Autodesk Fusion 360 part; units mm, degrees
(part 3 of 4)
  arc A61 (-18.7401, 17.7754) -> (-17.3539, 17.7855) centre (-18.0523, 18.5012) ccw
  line L30 (-18.7401, 17.7754) -> (-19.4311, 18.4301)
  spline S30 degree 5 poles (-19.4311, 18.4301) (-19.4412, 18.4397) (-19.4617, 18.4586) (-19.4931, 18.486) (-19.5364, 18.521) (-19.5924, 18.5625) (-19.6498, 18.6024) (-19.708, 18.6413) (-19.7667, 18.6797) (-19.8257, 18.7177) (-19.885, 18.7553) (-19.9448, 18.7924) (-20.0051, 18.8288) (-20.0661, 18.8644) (-20.1276, 18.8992) (-20.1898, 18.9332) (-20.2525, 18.9666) (-20.3156, 18.9995) (-20.379, 19.0319) (-20.4428, 19.0638) (-20.5069, 19.0953) (-20.5714, 19.1263) (-20.6362, 19.1568) (-20.7014, 19.1867) (-20.767, 19.2162) (-20.8329, 19.2451) (-20.8992, 19.2736) (-20.9657, 19.3016) (-21.0326, 19.3292) (-21.0998, 19.3564) (-21.1672, 19.3831) (-21.235, 19.4094) (-21.303, 19.4353) (-21.3713, 19.4607) (-21.4399, 19.4857) (-21.5088, 19.5103) (-21.5779, 19.5345) (-21.6473, 19.5583) (-21.7169, 19.5816) (-21.7868, 19.6046) (-21.8569, 19.6271) (-21.9273, 19.6493) (-21.9979, 19.6711) (-22.0687, 19.6925) (-22.1398, 19.7135) (-22.2111, 19.7341) (-22.2826, 19.7543) (-22.3543, 19.7742) (-22.4263, 19.7936) (-22.4985, 19.8127) (-22.5708, 19.8315) (-22.6434, 19.8498) (-22.7162, 19.8678) (-22.7892, 19.8854) (-22.8623, 19.9027) (-22.9357, 19.9195) (-23.0093, 19.9361) (-23.083, 19.9522) (-23.157, 19.968) (-23.2311, 19.9835) (-23.3054, 19.9986) (-23.3799, 20.0133) (-23.4545, 20.0277) (-23.5293, 20.0417) (-23.6043, 20.0554) (-23.6795, 20.0687) (-23.7548, 20.0817) (-23.8303, 20.0943) (-23.906, 20.1066) (-23.9818, 20.1185) (-24.0578, 20.1301) (-24.1187, 20.1391) (-24.1645, 20.1457) (-24.195, 20.1501) (-24.2103, 20.1522) knots 0 0 0 0 0 0 0.01428571 0.02857143 0.04285714 0.05714286 0.07142857 0.08571429 0.1 0.11428571 0.12857143 0.14285714 0.15714286 0.17142857 0.18571429 0.2 0.21428571 0.22857143 0.24285714 0.25714286 0.27142857 0.28571429 0.3 0.31428571 0.32857143 0.34285714 0.35714286 0.37142857 0.38571429 0.4 0.41428571 0.42857143 0.44285714 0.45714286 0.47142857 0.48571429 0.5 0.51428571 0.52857143 0.54285714 0.55714286 0.57142857 0.58571429 0.6 0.61428571 0.62857143 0.64285714 0.65714286 0.67142857 0.68571429 0.7 0.71428571 0.72857143 0.74285714 0.75714286 0.77142857 0.78571429 0.8 0.81428571 0.82857143 0.84285714 0.85714286 0.87142857 0.88571429 0.9 0.91428571 0.92857143 0.94285714 0.95714286 0.97142857 0.98571429 1 1 1 1 1 1
  arc A62 (-24.2103, 20.1522) -> (-25.4788, 18.5224) centre (0, 0) ccw
  spline S31 degree 5 poles (-22.6362, 14.3122) (-22.648, 14.3196) (-22.6713, 14.3348) (-22.7056, 14.3586) (-22.7502, 14.392) (-22.8041, 14.4361) (-22.8569, 14.4819) (-22.9089, 14.5288) (-22.9605, 14.5763) (-23.0118, 14.6241) (-23.0628, 14.6724) (-23.1135, 14.7212) (-23.1636, 14.7708) (-23.213, 14.8211) (-23.2619, 14.8723) (-23.3102, 14.9242) (-23.3579, 14.9767) (-23.4053, 15.0298) (-23.4522, 15.0834) (-23.4989, 15.1374) (-23.5451, 15.1918) (-23.591, 15.2467) (-23.6365, 15.302) (-23.6815, 15.3579) (-23.7262, 15.4142) (-23.7704, 15.471) (-23.8143, 15.5282) (-23.8578, 15.5859) (-23.901, 15.644) (-23.9438, 15.7024) (-23.9863, 15.7612) (-24.0284, 15.8205) (-24.0702, 15.88) (-24.1116, 15.94) (-24.1527, 16.0004) (-24.1934, 16.0611) (-24.2338, 16.1222) (-24.2739, 16.1836) (-24.3136, 16.2454) (-24.353, 16.3075) (-24.3921, 16.3699) (-24.4309, 16.4327) (-24.4693, 16.4958) (-24.5074, 16.5592) (-24.5452, 16.6229) (-24.5827, 16.687) (-24.6199, 16.7514) (-24.6567, 16.816) (-24.6933, 16.881) (-24.7295, 16.9463) (-24.7654, 17.0118) (-24.801, 17.0777) (-24.8363, 17.1438) (-24.8713, 17.2102) (-24.906, 17.2769) (-24.9404, 17.3439) (-24.9745, 17.4112) (-25.0082, 17.4787) (-25.0417, 17.5465) (-25.0749, 17.6146) (-25.1077, 17.6829) (-25.1403, 17.7515) (-25.1726, 17.8203) (-25.2045, 17.8894) (-25.2362, 17.9588) (-25.2676, 18.0283) (-25.2987, 18.0982) (-25.3294, 18.1683) (-25.3599, 18.2386) (-25.3901, 18.3092) (-25.42, 18.38) (-25.4437, 18.4368) (-25.4613, 18.4796) (-25.473, 18.5081) (-25.4788, 18.5224) knots 0 0 0 0 0 0 0.01428571 0.02857143 0.04285714 0.05714286 0.07142857 0.08571429 0.1 0.11428571 0.12857143 0.14285714 0.15714286 0.17142857 0.18571429 0.2 0.21428571 0.22857143 0.24285714 0.25714286 0.27142857 0.28571429 0.3 0.31428571 0.32857143 0.34285714 0.35714286 0.37142857 0.38571429 0.4 0.41428571 0.42857143 0.44285714 0.45714286 0.47142857 0.48571429 0.5 0.51428571 0.52857143 0.54285714 0.55714286 0.57142857 0.58571429 0.6 0.61428571 0.62857143 0.64285714 0.65714286 0.67142857 0.68571429 0.7 0.71428571 0.72857143 0.74285714 0.75714286 0.77142857 0.78571429 0.8 0.81428571 0.82857143 0.84285714 0.85714286 0.87142857 0.88571429 0.9 0.91428571 0.92857143 0.94285714 0.95714286 0.97142857 0.98571429 1 1 1 1 1 1
  line L31 (-22.6362, 14.3122) -> (-21.8319, 13.8031)
  arc A63 (-21.5014, 12.4568) -> (-21.8319, 13.8031) centre (-22.3667, 12.9581) ccw
  arc A64 (-21.5014, 12.4568) -> (-22.1886, 11.187) centre (0, 0) ccw
  arc A65 (-23.4964, 10.7273) -> (-22.1886, 11.187) centre (-23.0815, 11.6372) ccw
  line L32 (-23.4964, 10.7273) -> (-24.3625, 11.1222)
  spline S32 degree 5 poles (-24.3625, 11.1222) (-24.3752, 11.128) (-24.4007, 11.1392) (-24.4393, 11.155) (-24.4916, 11.174) (-24.5581, 11.1951) (-24.6253, 11.2142) (-24.693, 11.2321) (-24.761, 11.2493) (-24.8291, 11.2661) (-24.8974, 11.2824) (-24.966, 11.2981) (-25.0349, 11.3129) (-25.1041, 11.3268) (-25.1736, 11.3397) (-25.2435, 11.3517) (-25.3136, 11.363) (-25.3839, 11.3736) (-25.4545, 11.3836) (-25.5251, 11.3931) (-25.596, 11.4021) (-25.667, 11.4104) (-25.7382, 11.4182) (-25.8096, 11.4254) (-25.8812, 11.432) (-25.953, 11.438) (-26.0249, 11.4434) (-26.097, 11.4483) (-26.1692, 11.4527) (-26.2415, 11.4565) (-26.314, 11.4599) (-26.3866, 11.4628) (-26.4594, 11.4652) (-26.5322, 11.467) (-26.6052, 11.4684) (-26.6783, 11.4693) (-26.7516, 11.4697) (-26.8249, 11.4697) (-26.8984, 11.4692) (-26.9719, 11.4682) (-27.0456, 11.4668) (-27.1193, 11.4649) (-27.1932, 11.4626) (-27.2671, 11.4598) (-27.3412, 11.4566) (-27.4153, 11.4529) (-27.4895, 11.4488) (-27.5638, 11.4443) (-27.6382, 11.4394) (-27.7126, 11.434) (-27.7871, 11.4282) (-27.8617, 11.422) (-27.9364, 11.4154) (-28.0112, 11.4083) (-28.086, 11.4009) (-28.1608, 11.393) (-28.2358, 11.3848) (-28.3108, 11.3761) (-28.3859, 11.3671) (-28.461, 11.3576) (-28.5361, 11.3477) (-28.6114, 11.3375) (-28.6867, 11.3269) (-28.762, 11.3158) (-28.8374, 11.3044) (-28.9128, 11.2926) (-28.9883, 11.2804) (-29.0638, 11.2678) (-29.1393, 11.2549) (-29.2149, 11.2416) (-29.2905, 11.2279) (-29.3511, 11.2166) (-29.3965, 11.208) (-29.4268, 11.2022) (-29.4419, 11.1992) knots 0 0 0 0 0 0 0.01428571 0.02857143 0.04285714 0.05714286 0.07142857 0.08571429 0.1 0.11428571 0.12857143 0.14285714 0.15714286 0.17142857 0.18571429 0.2 0.21428571 0.22857143 0.24285714 0.25714286 0.27142857 0.28571429 0.3 0.31428571 0.32857143 0.34285714 0.35714286 0.37142857 0.38571429 0.4 0.41428571 0.42857143 0.44285714 0.45714286 0.47142857 0.48571429 0.5 0.51428571 0.52857143 0.54285714 0.55714286 0.57142857 0.58571429 0.6 0.61428571 0.62857143 0.64285714 0.65714286 0.67142857 0.68571429 0.7 0.71428571 0.72857143 0.74285714 0.75714286 0.77142857 0.78571429 0.8 0.81428571 0.82857143 0.84285714 0.85714286 0.87142857 0.88571429 0.9 0.91428571 0.92857143 0.94285714 0.95714286 0.97142857 0.98571429 1 1 1 1 1 1
  arc A66 (-29.4419, 11.1992) -> (-30.1125, 9.2458) centre (0, 0) ccw
  spline S33 degree 5 poles (-26.0568, 6.1867) (-26.0704, 6.19) (-26.0974, 6.1968) (-26.1376, 6.2081) (-26.1906, 6.2252) (-26.2559, 6.2494) (-26.3207, 6.2756) (-26.3851, 6.3031) (-26.4493, 6.3312) (-26.5134, 6.3598) (-26.5774, 6.3889) (-26.6411, 6.4187) (-26.7046, 6.4492) (-26.7677, 6.4808) (-26.8305, 6.5133) (-26.893, 6.5467) (-26.9553, 6.5809) (-27.0173, 6.6158) (-27.0791, 6.6512) (-27.1407, 6.6871) (-27.2021, 6.7236) (-27.2633, 6.7606) (-27.3243, 6.7982) (-27.3851, 6.8364) (-27.4456, 6.8751) (-27.5059, 6.9145) (-27.566, 6.9544) (-27.6259, 6.9948) (-27.6855, 7.0357) (-27.745, 7.0771) (-27.8043, 7.1189) (-27.8633, 7.1613) (-27.9222, 7.2041) (-27.9809, 7.2473) (-28.0393, 7.2911) (-28.0976, 7.3353) (-28.1556, 7.3799) (-28.2135, 7.425) (-28.2711, 7.4705) (-28.3285, 7.5165) (-28.3858, 7.5628) (-28.4428, 7.6096) (-28.4997, 7.6568) (-28.5563, 7.7044) (-28.6128, 7.7524) (-28.669, 7.8009) (-28.7251, 7.8497) (-28.7809, 7.8989) (-28.8366, 7.9484) (-28.892, 7.9984) (-28.9473, 8.0488) (-29.0024, 8.0995) (-29.0572, 8.1506) (-29.1119, 8.202) (-29.1663, 8.2539) (-29.2206, 8.306) (-29.2747, 8.3586) (-29.3285, 8.4115) (-29.3822, 8.4647) (-29.4357, 8.5184) (-29.489, 8.5723) (-29.542, 8.6266) (-29.5949, 8.6812) (-29.6476, 8.7362) (-29.7, 8.7915) (-29.7523, 8.8472) (-29.8044, 8.9031) (-29.8563, 8.9594) (-29.9079, 9.016) (-29.9594, 9.073) (-30.0107, 9.1303) (-30.0515, 9.1763) (-30.0821, 9.211) (-30.1024, 9.2342) (-30.1125, 9.2458) knots 0 0 0 0 0 0 0.01428571 0.02857143 0.04285714 0.05714286 0.07142857 0.08571429 0.1 0.11428571 0.12857143 0.14285714 0.15714286 0.17142857 0.18571429 0.2 0.21428571 0.22857143 0.24285714 0.25714286 0.27142857 0.28571429 0.3 0.31428571 0.32857143 0.34285714 0.35714286 0.37142857 0.38571429 0.4 0.41428571 0.42857143 0.44285714 0.45714286 0.47142857 0.48571429 0.5 0.51428571 0.52857143 0.54285714 0.55714286 0.57142857 0.58571429 0.6 0.61428571 0.62857143 0.64285714 0.65714286 0.67142857 0.68571429 0.7 0.71428571 0.72857143 0.74285714 0.75714286 0.77142857 0.78571429 0.8 0.81428571 0.82857143 0.84285714 0.85714286 0.87142857 0.88571429 0.9 0.91428571 0.92857143 0.94285714 0.95714286 0.97142857 0.98571429 1 1 1 1 1 1
  line L33 (-26.0568, 6.1867) -> (-25.1308, 5.9664)
  arc A67 (-24.3811, 4.8004) -> (-25.1308, 5.9664) centre (-25.3623, 4.9935) ccw
  arc A68 (-24.3811, 4.8004) -> (-24.6188, 3.3763) centre (0, 0) ccw
  arc A69 (-25.7064, 2.5168) -> (-24.6188, 3.3763) centre (-25.6095, 3.5121) ccw
  line L34 (-25.7064, 2.5168) -> (-26.6538, 2.6091)
  spline S34 degree 5 poles (-26.6538, 2.6091) (-26.6677, 2.6105) (-26.6955, 2.6128) (-26.7371, 2.6152) (-26.7928, 2.6162) (-26.8625, 2.6145) (-26.9323, 2.6108) (-27.0021, 2.6057) (-27.072, 2.5999) (-27.1419, 2.5937) (-27.2118, 2.5869) (-27.2818, 2.5795) (-27.3517, 2.5711) (-27.4217, 2.5618) (-27.4916, 2.5514) (-27.5616, 2.5401) (-27.6316, 2.528) (-27.7016, 2.5152) (-27.7715, 2.5018) (-27.8415, 2.4878) (-27.9114, 2.4733) (-27.9813, 2.4581) (-28.0512, 2.4424) (-28.121, 2.426) (-28.1909, 2.4089) (-28.2607, 2.3913) (-28.3305, 2.3731) (-28.4002, 2.3543) (-28.4699, 2.335) (-28.5396, 2.3152) (-28.6093, 2.2948) (-28.6789, 2.274) (-28.7485, 2.2526) (-28.818, 2.2307) (-28.8875, 2.2083) (-28.9569, 2.1854) (-29.0263, 2.162) (-29.0957, 2.1382) (-29.165, 2.1138) (-29.2342, 2.089) (-29.3034, 2.0638) (-29.3726, 2.0381) (-29.4417, 2.0119) (-29.5107, 1.9852) (-29.5797, 1.9582) (-29.6486, 1.9306) (-29.7175, 1.9027) (-29.7863, 1.8743) (-29.855, 1.8454) (-29.9237, 1.8162) (-29.9923, 1.7865) (-30.0608, 1.7564) (-30.1293, 1.7259) (-30.1977, 1.695) (-30.2661, 1.6637) (-30.3343, 1.6319) (-30.4025, 1.5998) (-30.4707, 1.5672) (-30.5387, 1.5343) (-30.6067, 1.5009) (-30.6746, 1.4672) (-30.7424, 1.4331) (-30.8102, 1.3986) (-30.8778, 1.3637) (-30.9454, 1.3284) (-31.0129, 1.2928) (-31.0803, 1.2567) (-31.1477, 1.2203) (-31.2149, 1.1836) (-31.2821, 1.1464) (-31.3492, 1.1089) (-31.4028, 1.0786) (-31.4429, 1.0557) (-31.4697, 1.0404) (-31.4831, 1.0327) knots 0 0 0 0 0 0 0.01428571 0.02857143 0.04285714 0.05714286 0.07142857 0.08571429 0.1 0.11428571 0.12857143 0.14285714 0.15714286 0.17142857 0.18571429 0.2 0.21428571 0.22857143 0.24285714 0.25714286 0.27142857 0.28571429 0.3 0.31428571 0.32857143 0.34285714 0.35714286 0.37142857 0.38571429 0.4 0.41428571 0.42857143 0.44285714 0.45714286 0.47142857 0.48571429 0.5 0.51428571 0.52857143 0.54285714 0.55714286 0.57142857 0.58571429 0.6 0.61428571 0.62857143 0.64285714 0.65714286 0.67142857 0.68571429 0.7 0.71428571 0.72857143 0.74285714 0.75714286 0.77142857 0.78571429 0.8 0.81428571 0.82857143 0.84285714 0.85714286 0.87142857 0.88571429 0.9 0.91428571 0.92857143 0.94285714 0.95714286 0.97142857 0.98571429 1 1 1 1 1 1
  arc A70 (-31.4831, 1.0327) -> (-31.4831, -1.0327) centre (0, 0) ccw
  spline S35 degree 5 poles (-26.6538, -2.6091) (-26.6677, -2.6105) (-26.6955, -2.6128) (-26.7371, -2.6152) (-26.7928, -2.6162) (-26.8625, -2.6145) (-26.9323, -2.6108) (-27.0021, -2.6057) (-27.072, -2.5999) (-27.1419, -2.5937) (-27.2118, -2.5869) (-27.2818, -2.5795) (-27.3517, -2.5711) (-27.4217, -2.5618) (-27.4916, -2.5514) (-27.5616, -2.5401) (-27.6316, -2.528) (-27.7016, -2.5152) (-27.7715, -2.5018) (-27.8415, -2.4878) (-27.9114, -2.4733) (-27.9813, -2.4581) (-28.0512, -2.4424) (-28.121, -2.426) (-28.1909, -2.4089) (-28.2607, -2.3913) (-28.3305, -2.3731) (-28.4002, -2.3543) (-28.4699, -2.335) (-28.5396, -2.3152) (-28.6093, -2.2948) (-28.6789, -2.274) (-28.7485, -2.2526) (-28.818, -2.2307) (-28.8875, -2.2083) (-28.9569, -2.1854) (-29.0263, -2.162) (-29.0957, -2.1382) (-29.165, -2.1138) (-29.2342, -2.089) (-29.3034, -2.0638) (-29.3726, -2.0381) (-29.4417, -2.0119) (-29.5107, -1.9852) (-29.5797, -1.9582) (-29.6486, -1.9306) (-29.7175, -1.9027) (-29.7863, -1.8743) (-29.855, -1.8454) (-29.9237, -1.8162) (-29.9923, -1.7865) (-30.0608, -1.7564) (-30.1293, -1.7259) (-30.1977, -1.695) (-30.2661, -1.6637) (-30.3343, -1.6319) (-30.4025, -1.5998) (-30.4707, -1.5672) (-30.5387, -1.5343) (-30.6067, -1.5009) (-30.6746, -1.4672) (-30.7424, -1.4331) (-30.8102, -1.3986) (-30.8778, -1.3637) (-30.9454, -1.3284) (-31.0129, -1.2928) (-31.0803, -1.2567) (-31.1477, -1.2203) (-31.2149, -1.1836) (-31.2821, -1.1464) (-31.3492, -1.1089) (-31.4028, -1.0786) (-31.4429, -1.0557) (-31.4697, -1.0404) (-31.4831, -1.0327) knots 0 0 0 0 0 0 0.01428571 0.02857143 0.04285714 0.05714286 0.07142857 0.08571429 0.1 0.11428571 0.12857143 0.14285714 0.15714286 0.17142857 0.18571429 0.2 0.21428571 0.22857143 0.24285714 0.25714286 0.27142857 0.28571429 0.3 0.31428571 0.32857143 0.34285714 0.35714286 0.37142857 0.38571429 0.4 0.41428571 0.42857143 0.44285714 0.45714286 0.47142857 0.48571429 0.5 0.51428571 0.52857143 0.54285714 0.55714286 0.57142857 0.58571429 0.6 0.61428571 0.62857143 0.64285714 0.65714286 0.67142857 0.68571429 0.7 0.71428571 0.72857143 0.74285714 0.75714286 0.77142857 0.78571429 0.8 0.81428571 0.82857143 0.84285714 0.85714286 0.87142857 0.88571429 0.9 0.91428571 0.92857143 0.94285714 0.95714286 0.97142857 0.98571429 1 1 1 1 1 1
  line L35 (-26.6538, -2.6091) -> (-25.7064, -2.5168)
  arc A71 (-24.6188, -3.3763) -> (-25.7064, -2.5168) centre (-25.6095, -3.5121) ccw
  arc A72 (-24.6188, -3.3763) -> (-24.3811, -4.8004) centre (0, 0) ccw
  arc A73 (-25.1308, -5.9664) -> (-24.3811, -4.8004) centre (-25.3623, -4.9935) ccw
  line L36 (-25.1308, -5.9664) -> (-26.0568, -6.1867)
  spline S36 degree 5 poles (-26.0568, -6.1867) (-26.0704, -6.19) (-26.0974, -6.1968) (-26.1376, -6.2081) (-26.1906, -6.2252) (-26.2559, -6.2494) (-26.3207, -6.2756) (-26.3851, -6.3031) (-26.4493, -6.3312) (-26.5134, -6.3598) (-26.5774, -6.3889) (-26.6411, -6.4187) (-26.7046, -6.4492) (-26.7677, -6.4808) (-26.8305, -6.5133) (-26.893, -6.5467) (-26.9553, -6.5809) (-27.0173, -6.6158) (-27.0791, -6.6512) (-27.1407, -6.6871) (-27.2021, -6.7236) (-27.2633, -6.7606) (-27.3243, -6.7982) (-27.3851, -6.8364) (-27.4456, -6.8751) (-27.5059, -6.9145) (-27.566, -6.9544) (-27.6259, -6.9948) (-27.6855, -7.0357) (-27.745, -7.0771) (-27.8043, -7.1189) (-27.8633, -7.1613) (-27.9222, -7.2041) (-27.9809, -7.2473) (-28.0393, -7.2911) (-28.0976, -7.3353) (-28.1556, -7.3799) (-28.2135, -7.425) (-28.2711, -7.4705) (-28.3285, -7.5165) (-28.3858, -7.5628) (-28.4428, -7.6096) (-28.4997, -7.6568) (-28.5563, -7.7044) (-28.6128, -7.7524) (-28.669, -7.8009) (-28.7251, -7.8497) (-28.7809, -7.8989) (-28.8366, -7.9484) (-28.892, -7.9984) (-28.9473, -8.0488) (-29.0024, -8.0995) (-29.0572, -8.1506) (-29.1119, -8.202) (-29.1663, -8.2539) (-29.2206, -8.306) (-29.2747, -8.3586) (-29.3285, -8.4115) (-29.3822, -8.4647) (-29.4357, -8.5184) (-29.489, -8.5723) (-29.542, -8.6266) (-29.5949, -8.6812) (-29.6476, -8.7362) (-29.7, -8.7915) (-29.7523, -8.8472) (-29.8044, -8.9031) (-29.8563, -8.9594) (-29.9079, -9.016) (-29.9594, -9.073) (-30.0107, -9.1303) (-30.0515, -9.1763) (-30.0821, -9.211) (-30.1024, -9.2342) (-30.1125, -9.2458) knots 0 0 0 0 0 0 0.01428571 0.02857143 0.04285714 0.05714286 0.07142857 0.08571429 0.1 0.11428571 0.12857143 0.14285714 0.15714286 0.17142857 0.18571429 0.2 0.21428571 0.22857143 0.24285714 0.25714286 0.27142857 0.28571429 0.3 0.31428571 0.32857143 0.34285714 0.35714286 0.37142857 0.38571429 0.4 0.41428571 0.42857143 0.44285714 0.45714286 0.47142857 0.48571429 0.5 0.51428571 0.52857143 0.54285714 0.55714286 0.57142857 0.58571429 0.6 0.61428571 0.62857143 0.64285714 0.65714286 0.67142857 0.68571429 0.7 0.71428571 0.72857143 0.74285714 0.75714286 0.77142857 0.78571429 0.8 0.81428571 0.82857143 0.84285714 0.85714286 0.87142857 0.88571429 0.9 0.91428571 0.92857143 0.94285714 0.95714286 0.97142857 0.98571429 1 1 1 1 1 1
  arc A74 (-30.1125, -9.2458) -> (-29.4419, -11.1992) centre (0, 0) ccw
  spline S37 degree 5 poles (-24.3625, -11.1222) (-24.3752, -11.128) (-24.4007, -11.1392) (-24.4393, -11.155) (-24.4916, -11.174) (-24.5581, -11.1951) (-24.6253, -11.2142) (-24.693, -11.2321) (-24.761, -11.2493) (-24.8291, -11.2661) (-24.8974, -11.2824) (-24.966, -11.2981) (-25.0349, -11.3129) (-25.1041, -11.3268) (-25.1736, -11.3397) (-25.2435, -11.3517) (-25.3136, -11.363) (-25.3839, -11.3736) (-25.4545, -11.3836) (-25.5251, -11.3931) (-25.596, -11.4021) (-25.667, -11.4104) (-25.7382, -11.4182) (-25.8096, -11.4254) (-25.8812, -11.432) (-25.953, -11.438) (-26.0249, -11.4434) (-26.097, -11.4483) (-26.1692, -11.4527) (-26.2415, -11.4565) (-26.314, -11.4599) (-26.3866, -11.4628) (-26.4594, -11.4652) (-26.5322, -11.467) (-26.6052, -11.4684) (-26.6783, -11.4693) (-26.7516, -11.4697) (-26.8249, -11.4697) (-26.8984, -11.4692) (-26.9719, -11.4682) (-27.0456, -11.4668) (-27.1193, -11.4649) (-27.1932, -11.4626) (-27.2671, -11.4598) (-27.3412, -11.4566) (-27.4153, -11.4529) (-27.4895, -11.4488) (-27.5638, -11.4443) (-27.6382, -11.4394) (-27.7126, -11.434) (-27.7871, -11.4282) (-27.8617, -11.422) (-27.9364, -11.4154) (-28.0112, -11.4083) (-28.086, -11.4009) (-28.1608, -11.393) (-28.2358, -11.3848) (-28.3108, -11.3761) (-28.3859, -11.3671) (-28.461, -11.3576) (-28.5361, -11.3477) (-28.6114, -11.3375) (-28.6867, -11.3269) (-28.762, -11.3158) (-28.8374, -11.3044) (-28.9128, -11.2926) (-28.9883, -11.2804) (-29.0638, -11.2678) (-29.1393, -11.2549) (-29.2149, -11.2416) (-29.2905, -11.2279) (-29.3511, -11.2166) (-29.3965, -11.208) (-29.4268, -11.2022) (-29.4419, -11.1992) knots 0 0 0 0 0 0 0.01428571 0.02857143 0.04285714 0.05714286 0.07142857 0.08571429 0.1 0.11428571 0.12857143 0.14285714 0.15714286 0.17142857 0.18571429 0.2 0.21428571 0.22857143 0.24285714 0.25714286 0.27142857 0.28571429 0.3 0.31428571 0.32857143 0.34285714 0.35714286 0.37142857 0.38571429 0.4 0.41428571 0.42857143 0.44285714 0.45714286 0.47142857 0.48571429 0.5 0.51428571 0.52857143 0.54285714 0.55714286 0.57142857 0.58571429 0.6 0.61428571 0.62857143 0.64285714 0.65714286 0.67142857 0.68571429 0.7 0.71428571 0.72857143 0.74285714 0.75714286 0.77142857 0.78571429 0.8 0.81428571 0.82857143 0.84285714 0.85714286 0.87142857 0.88571429 0.9 0.91428571 0.92857143 0.94285714 0.95714286 0.97142857 0.98571429 1 1 1 1 1 1
  line L37 (-24.3625, -11.1222) -> (-23.4964, -10.7273)
  arc A75 (-22.1886, -11.187) -> (-23.4964, -10.7273) centre (-23.0815, -11.6372) ccw
  arc A76 (-22.1886, -11.187) -> (-21.5014, -12.4568) centre (0, 0) ccw
  circle A77 centre (0, 15) radius 2.5
  circle A78 centre (-10.6066, 10.6066) radius 2.5
  circle A79 centre (-15, 0) radius 2.5
  circle A80 centre (-10.6066, -10.6066) radius 2.5
  circle A81 centre (0, -15) radius 2.5
  circle A82 centre (10.6066, -10.6066) radius 2.5
  circle A83 centre (15, 0) radius 2.5
  circle A84 centre (10.6066, 10.6066) radius 2.5
  dimension "d29" = 5
  dimension "d30" = 15
  dimension "d32" = 360
  measures "d29" diameter of A77
  measures "d30" distance of A77.centre A0.centre
component "Spur Gear (19 teeth)" placed x (1, 0, 0) y (0, 1, 0) z (0, 0, 1) at (0, 0, 0)

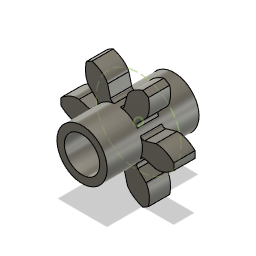
design "gear(small)right"
description: small size, for right
description: Spur Gear; Module: 2.0; Num Teeth: 6; Pressure Angle: 20.0; Backlash: 0.00 mm
Autodesk Fusion 360 part; units mm, degrees
sketch "草图1" plane through (0, 0, 0) normal (0, 0, 1) x (1, 0, 0) in component "Spur Gear (6 teeth)"
  circle A0 centre (0, 0) radius 3.5492
  circle A1 centre (0, 0) radius 2.5
extrude "拉伸1" add sketch "草图1" along normal blind 8 and the other way blind 5 in component "Spur Gear (6 teeth)"
sketch "草图2" plane through (0, 0, 0) normal (0, 0, 1) x (1, 0, 0) in component "Spur Gear (6 teeth)"
  spline S0 degree 5 poles (5.4237, -1.5403) (5.4306, -1.5422) (5.4444, -1.5458) (5.4654, -1.5503) (5.4937, -1.5547) (5.5295, -1.5577) (5.5656, -1.5592) (5.602, -1.5596) (5.6385, -1.5595) (5.6751, -1.559) (5.7117, -1.558) (5.7485, -1.5565) (5.7854, -1.5541) (5.8224, -1.5509) (5.8596, -1.5469) (5.8968, -1.542) (5.9342, -1.5365) (5.9716, -1.5304) (6.009, -1.5238) (6.0465, -1.5167) (6.084, -1.509) (6.1216, -1.5009) (6.1592, -1.4921) (6.1968, -1.4828) (6.2344, -1.473) (6.2721, -1.4625) (6.3098, -1.4516) (6.3475, -1.4402) (6.3851, -1.4282) (6.4228, -1.4158) (6.4605, -1.403) (6.4982, -1.3896) (6.5358, -1.3757) (6.5734, -1.3614) (6.611, -1.3466) (6.6486, -1.3313) (6.6861, -1.3156) (6.7236, -1.2994) (6.7611, -1.2828) (6.7985, -1.2657) (6.8359, -1.2482) (6.8732, -1.2302) (6.9104, -1.2118) (6.9476, -1.193) (6.9848, -1.1737) (7.0219, -1.154) (7.0589, -1.1339) (7.0958, -1.1133) (7.1326, -1.0923) (7.1694, -1.071) (7.2061, -1.0492) (7.2427, -1.027) (7.2792, -1.0043) (7.3157, -0.9813) (7.352, -0.9579) (7.3882, -0.9341) (7.4244, -0.9098) (7.4604, -0.8852) (7.4963, -0.8602) (7.5321, -0.8348) (7.5678, -0.809) (7.6034, -0.7828) (7.6388, -0.7563) (7.6742, -0.7293) (7.7094, -0.702) (7.7445, -0.6743) (7.7794, -0.6462) (7.8142, -0.6178) (7.8489, -0.589) (7.8834, -0.5598) (7.9178, -0.5303) (7.9452, -0.5063) (7.9657, -0.4882) (7.9794, -0.4761) (7.9862, -0.47) knots 0 0 0 0 0 0 0.01428571 0.02857143 0.04285714 0.05714286 0.07142857 0.08571429 0.1 0.11428571 0.12857143 0.14285714 0.15714286 0.17142857 0.18571429 0.2 0.21428571 0.22857143 0.24285714 0.25714286 0.27142857 0.28571429 0.3 0.31428571 0.32857143 0.34285714 0.35714286 0.37142857 0.38571429 0.4 0.41428571 0.42857143 0.44285714 0.45714286 0.47142857 0.48571429 0.5 0.51428571 0.52857143 0.54285714 0.55714286 0.57142857 0.58571429 0.6 0.61428571 0.62857143 0.64285714 0.65714286 0.67142857 0.68571429 0.7 0.71428571 0.72857143 0.74285714 0.75714286 0.77142857 0.78571429 0.8 0.81428571 0.82857143 0.84285714 0.85714286 0.87142857 0.88571429 0.9 0.91428571 0.92857143 0.94285714 0.95714286 0.97142857 0.98571429 1 1 1 1 1 1
  spline S1 degree 5 poles (5.4237, 1.5403) (5.4306, 1.5422) (5.4444, 1.5458) (5.4654, 1.5503) (5.4937, 1.5547) (5.5295, 1.5577) (5.5656, 1.5592) (5.602, 1.5596) (5.6385, 1.5595) (5.6751, 1.559) (5.7117, 1.558) (5.7485, 1.5565) (5.7854, 1.5541) (5.8224, 1.5509) (5.8596, 1.5469) (5.8968, 1.542) (5.9342, 1.5365) (5.9716, 1.5304) (6.009, 1.5238) (6.0465, 1.5167) (6.084, 1.509) (6.1216, 1.5009) (6.1592, 1.4921) (6.1968, 1.4828) (6.2344, 1.473) (6.2721, 1.4625) (6.3098, 1.4516) (6.3475, 1.4402) (6.3851, 1.4282) (6.4228, 1.4158) (6.4605, 1.403) (6.4982, 1.3896) (6.5358, 1.3757) (6.5734, 1.3614) (6.611, 1.3466) (6.6486, 1.3313) (6.6861, 1.3156) (6.7236, 1.2994) (6.7611, 1.2828) (6.7985, 1.2657) (6.8359, 1.2482) (6.8732, 1.2302) (6.9104, 1.2118) (6.9476, 1.193) (6.9848, 1.1737) (7.0219, 1.154) (7.0589, 1.1339) (7.0958, 1.1133) (7.1326, 1.0923) (7.1694, 1.071) (7.2061, 1.0492) (7.2427, 1.027) (7.2792, 1.0043) (7.3157, 0.9813) (7.352, 0.9579) (7.3882, 0.9341) (7.4244, 0.9098) (7.4604, 0.8852) (7.4963, 0.8602) (7.5321, 0.8348) (7.5678, 0.809) (7.6034, 0.7828) (7.6388, 0.7563) (7.6742, 0.7293) (7.7094, 0.702) (7.7445, 0.6743) (7.7794, 0.6462) (7.8142, 0.6178) (7.8489, 0.589) (7.8834, 0.5598) (7.9178, 0.5303) (7.9452, 0.5063) (7.9657, 0.4882) (7.9794, 0.4761) (7.9862, 0.47) knots 0 0 0 0 0 0 0.01428571 0.02857143 0.04285714 0.05714286 0.07142857 0.08571429 0.1 0.11428571 0.12857143 0.14285714 0.15714286 0.17142857 0.18571429 0.2 0.21428571 0.22857143 0.24285714 0.25714286 0.27142857 0.28571429 0.3 0.31428571 0.32857143 0.34285714 0.35714286 0.37142857 0.38571429 0.4 0.41428571 0.42857143 0.44285714 0.45714286 0.47142857 0.48571429 0.5 0.51428571 0.52857143 0.54285714 0.55714286 0.57142857 0.58571429 0.6 0.61428571 0.62857143 0.64285714 0.65714286 0.67142857 0.68571429 0.7 0.71428571 0.72857143 0.74285714 0.75714286 0.77142857 0.78571429 0.8 0.81428571 0.82857143 0.84285714 0.85714286 0.87142857 0.88571429 0.9 0.91428571 0.92857143 0.94285714 0.95714286 0.97142857 0.98571429 1 1 1 1 1 1
  arc A0 (7.9862, -0.47) -> (7.9862, 0.47) centre (0, 0) ccw
  line L0 (3.4046, -0.9696) -> (5.4237, -1.5403)
  line L1 (3.4046, 0.9696) -> (5.4237, 1.5403)
  line L2 (3.4046, -0.9696) -> (3.4046, 0.9696)
  point P0 (5.5935, -1.5594)
  point P1 (5.7697, -1.555)
  point P2 (5.9497, -1.5339)
  point P3 (6.1326, -1.4982)
  point P4 (6.3176, -1.4491)
  point P5 (6.5041, -1.3873)
  point P6 (6.6914, -1.3132)
  point P7 (6.8792, -1.2272)
  point P8 (7.0668, -1.1294)
  point P9 (7.2538, -1.02)
  point P10 (7.4397, -0.8993)
  point P11 (7.6241, -0.7673)
  point P12 (7.8064, -0.6241)
  point P13 (5.5935, 1.5594)
  point P14 (5.7697, 1.555)
  point P15 (5.9497, 1.5339)
  point P16 (6.1326, 1.4982)
  point P17 (6.3176, 1.4491)
  point P18 (6.5041, 1.3873)
  point P19 (6.6914, 1.3132)
  point P20 (6.8792, 1.2272)
  point P21 (7.0668, 1.1294)
  point P22 (7.2538, 1.02)
  point P23 (7.4397, 0.8993)
  point P24 (7.6241, 0.7673)
  point P25 (7.8064, 0.6241)
extrude "拉伸2" add sketch "草图2" along normal blind 3 in component "Spur Gear (6 teeth)"
fillet "圆角1" radius 0.5 2 edges at (3.4135, -0.9721, 1.5) (3.4135, 0.9721, 1.5) in component "Spur Gear (6 teeth)"
pattern_circular "C-阵列1" count 6 over 360 about axis through (0, 0, -5) along (0, 0, 1) of "拉伸2", "圆角1" in component "Spur Gear (6 teeth)"
sketch "草图3" plane through (0, 0, 0) normal (0, 0, 1) x (1, 0, 0) in component "Spur Gear (6 teeth)"
  circle A0 centre (0, 0) radius 6 construction
component "Spur Gear (6 teeth)" placed x (1, 0, 0) y (0, 1, 0) z (0, 0, 1) at (0, 0, 0)

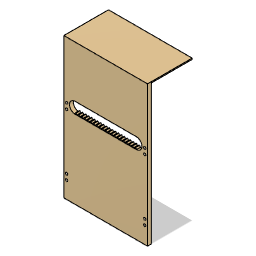
design "extension (left and right)"
Autodesk Fusion 360 part; units mm, degrees
sketch "Sketch1" plane through (0, 0, 0) normal (0, 1, 0) x (1, 0, 0)
  line L0 (0, 0) -> (0, -7)
  line L1 (0, -7) -> (-150, -7)
  line L2 (-150, -7) -> (-150, 0)
  line L3 (-150, 0) -> (0, 0)
  dimension "d1" = 7
  dimension "d2" = 150
  constraint coincident L0.start L3.end
  constraint vertical L0
  constraint perpendicular L0 L1
  constraint perpendicular L1 L2
  constraint perpendicular L0 L3
  measures "d1" distance of L0.start L0.end
  measures "d2" distance of L0.end L1.end
extrude "Extrude1" add sketch "Sketch1" against normal blind 252 makes body 1
sketch "Sketch2" plane through (0, 0, 0) normal (1, 0, 0) x (0, 0, -1)
  line L0 (0, 0) -> (73, 0)
  line L1 (73, 0) -> (73, -2)
  line L2 (73, -2) -> (0, -2)
  line L3 (0, -2) -> (0, 0)
  dimension "d5" = 73
  dimension "d6" = 2
  constraint horizontal L0
  constraint vertical L1
  constraint horizontal L2
  constraint vertical L3
  constraint coincident L0.start L3.end
  measures "d5" distance of L0.start L0.end
  measures "d6" distance of L2.end L0.start
extrude "Extrude2" add sketch "Sketch2" against normal blind 150 bodies 1
sketch "Sketch3" plane through (0, 0, 0) normal (0, 0, 1) x (1, 0, 0)
  circle A0 centre (-5, -112) radius 2.5
  circle A1 centre (-5, -102) radius 2.5
  line L0 (0, 0) -> (-150, 0)
  line L1 (0, 0) -> (0, -252)
  circle A2 centre (-145, -102) radius 2.5
  circle A3 centre (-145, -112) radius 2.5
  line L2 (-150, 0) -> (-150, -252)
  dimension "d9" = 102
  dimension "d10" = 10
  dimension "d11" = 5
  dimension "d12" = 5
  dimension "d71" = 5
  dimension "d72" = 5
  dimension "d73" = 5
  dimension "d74" = 10
  dimension "d75" = 5
  constraint horizontal A1.centre A2.centre
  constraint horizontal A0.centre A3.centre
  constraint vertical A2.centre A3.centre
  measures "d9" distance of A1.centre L0
  measures "d10" distance of A0.centre A1.centre
  measures "d11" diameter of A0
  measures "d12" diameter of A1
  measures "d16" radius of L0.end
  measures "d71" distance of A1.centre L1
  measures "d72" diameter of A2
  measures "d73" diameter of A3
  measures "d74" distance of A2.centre A3.centre
  measures "d75" distance of A2.centre L2
sketch "Sketch4" plane through (0, 0, 7) normal (0, 0, 1) x (1, 0, 0)
  line L0 (0, 0) -> (-150, 0)
  line L1 (-150, 0) -> (-150, -252)
  line L2 (-150, -252) -> (0, -252)
  line L3 (0, -252) -> (0, 0)
  line L4 (-130, -92) -> (-20, -92)
  line L5 (-130, -112) -> (-20, -112)
  arc A0 (-130, -92) -> (-130, -112) centre (-130, -102) ccw
  arc A1 (-20, -112) -> (-20, -92) centre (-20, -102) ccw
  point P0 (-5, -102)
  point P1 (-5, -112)
  dimension "d13" = 102
  dimension "d14" = 20
  dimension "d15" = 10
  dimension "d16" = 10
  dimension "d17" = 110
  dimension "d18" = 20
  dimension "d59" = 150
  constraint perpendicular L1 L4
  constraint perpendicular L1 L5
  constraint tangent L5 A0
  constraint tangent L4 A0
  constraint tangent L5 A1
  constraint tangent L4 A1
  measures "d13" vertical distance of L0.start A0.centre
  measures "d14" distance of L4 L5
  measures "d15" radius of A0
  measures "d16" radius of A1
  measures "d17" distance of L4.start L4.end
  measures "d18" horizontal distance of L0.start L4.end
  measures "d59" distance of L0.start L0.end
extrude "Extrude6" cut sketch "Sketch4" against normal blind 100 contours L4 L5 A0 A1 bodies 1
sketch "草图6" plane through (0, 0, 7) normal (0, 0, 1) x (1, 0, 0)
  line L0 (-20, -112) -> (-130, -112)
  arc A0 (-130, -92) -> (-130, -112) centre (-130, -102) ccw
  line L1 (-130, -92) -> (-20, -92)
  arc A1 (-20, -112) -> (-20, -92) centre (-20, -102) ccw
  line L2 (0, 0) -> (-150, 0)
  line L3 (-150, 0) -> (-150, -252)
  line L4 (-150, -252) -> (0, -252)
  line L5 (0, -252) -> (0, 0)
  line L6 (-130, -112) -> (-128.9739, -109.1809)
  line L7 (-130, -112) -> (-125.5798, -112) construction
  line L8 (-128.9739, -109.1809) -> (-127.9739, -109.1809)
  line L9 (-127.9739, -109.1809) -> (-126.9479, -112)
  line L10 (-127.9739, -109.1809) -> (-122.2899, -109.1809) construction
  line L11 (-130, -112) -> (-126.9479, -112)
  dimension "d43" = 3
  dimension "d44" = 70
  dimension "d45" = 1
  dimension "d46" = 70
  dimension "d47" = 3
  constraint horizontal L7
  constraint coincident L0.end A0.end
  constraint horizontal L8
  constraint horizontal L10
  measures "d43" distance of L0.end L6.end
  measures "d44" angle of L6 L7
  measures "d45" distance of L6.end L8.end
  measures "d46" angle of L9 L10
  measures "d47" distance of L8.end L9.end
extrude "拉伸7" add sketch "草图6" against normal blind 7 separate body contours L0 L6 L8 L9 L11 makes body 2
pattern_linear "R-阵列2" count 21 spacing 5.35 along (1, 0, 0) of "拉伸7" makes body 3 at (-122.6153, -112, 2.3333) makes body 4 at (-117.2653, -112, 2.3333) makes body 5 at (-111.9153, -112, 2.3333) makes body 6 at (-106.5653, -112, 2.3333) makes body 7 at (-95.8653, -112, 2.3333) makes body 8 at (-90.5153, -112, 2.3333) makes body 9 at (-85.1653, -112, 2.3333) makes body 10 at (-69.1153, -112, 2.3333) makes body 11 at (-101.2153, -112, 2.3333) makes body 12 at (-79.8153, -112, 2.3333) makes body 13 at (-74.4653, -112, 2.3333) makes body 14 at (-63.7653, -112, 2.3333) makes body 15 at (-58.4153, -112, 2.3333) makes body 16 at (-53.0653, -112, 2.3333) makes body 17 at (-47.7153, -112, 2.3333) makes body 18 at (-42.3653, -112, 2.3333) makes body 19 at (-37.0153, -112, 2.3333) makes body 20 at (-31.6653, -112, 2.3333) makes body 21 at (-26.3153, -112, 2.3333) makes body 22 at (-20.9653, -112, 2.3333)
sketch "草图7" plane through (0, 0, 7) normal (0, 0, 1) x (1, 0, 0)
  line L0 (-20, -112) -> (-130, -112)
  arc A0 (-130, -92) -> (-130, -112) centre (-130, -102) ccw
  line L1 (-130, -92) -> (-20, -92)
  arc A1 (-20, -112) -> (-20, -92) centre (-20, -102) ccw
  line L2 (0, 0) -> (-150, 0)
  line L3 (-150, 0) -> (-150, -252)
  line L4 (-150, -252) -> (0, -252)
  line L5 (0, -252) -> (0, 0)
  circle A2 centre (-5, -222) radius 2.5
  circle A3 centre (-5, -212) radius 2.5
  circle A4 centre (-145, -222) radius 2.5
  circle A5 centre (-145, -212) radius 2.5
  dimension "d60" = 5
  dimension "d61" = 5
  dimension "d62" = 5
  dimension "d63" = 5
  dimension "d64" = 10
  dimension "d65" = 30
  dimension "d66" = 5
  dimension "d67" = 5
  dimension "d68" = 5
  dimension "d69" = 5
  constraint horizontal A2.centre A4.centre
  constraint horizontal A3.centre A5.centre
  measures "d60" diameter of A2
  measures "d61" diameter of A3
  measures "d62" distance of L5 A2.centre
  measures "d63" distance of L5 A3.centre
  measures "d64" distance of A2.centre A3.centre
  measures "d65" distance of L4 A2.centre
  measures "d66" diameter of A4
  measures "d67" diameter of A5
  measures "d68" distance of L3 A4.centre
  measures "d69" distance of L3 A5.centre
extrude "拉伸8" cut sketch "草图7" against normal through all contours A2 | A3 | A4 | A5 bodies 1
extrude "拉伸9" cut sketch "Sketch3" along normal through all bodies 1
thread "螺纹1" "ISO Metric profile 5.0 M5x0.8 6H" major diameter 5.12 minor diameter 4.234 pitch 0.8 angle 60 resizes the face on face at (-144.2038, -209.6302, 2.3333) on bodies 1
thread "螺纹2" "ISO Metric profile 5.0 M5x0.8 6H" major diameter 5.12 minor diameter 4.234 pitch 0.8 angle 60 resizes the face on face at (-145.6771, -219.5934, 4.6667) on bodies 1
thread "螺纹3" "ISO Metric profile 5.0 M5x0.8 6H" major diameter 5.12 minor diameter 4.234 pitch 0.8 angle 60 resizes the face on face at (-2.5773, -212.6169, 4.6667) on bodies 1
thread "螺纹4" "ISO Metric profile 5.0 M5x0.8 6H" major diameter 5.12 minor diameter 4.234 pitch 0.8 angle 60 resizes the face on face at (-7.4227, -222.6169, 2.3333) on bodies 1
thread "螺纹5" "ISO Metric profile 5.0 M5x0.8 6H" major diameter 5.12 minor diameter 4.234 pitch 0.8 angle 60 resizes the face on face at (-144.2038, -99.6302, 2.3333) on face at (-144.2038, -109.6302, 2.3333) on face at (-7.3492, -111.1449, 4.6667) on face at (-7.3492, -101.1449, 4.6667) on bodies 1

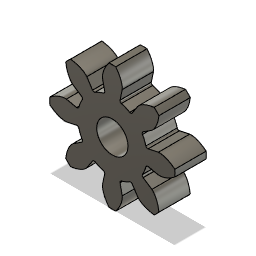
design "gear for left"
description: middle size
description: Spur Gear; Module: 2.0; Num Teeth: 8; Pressure Angle: 20.0; Backlash: 0.00 mm
Autodesk Fusion 360 part; units mm, degrees
sketch "草图1" plane through (0, 0, 0) normal (0, 0, 1) x (1, 0, 0) in component "Spur Gear (8 teeth)"
  circle A0 centre (0, 0) radius 5.5492
  circle A1 centre (0, 0) radius 2.5
extrude "拉伸1" add sketch "草图1" along normal blind 5 and the other way blind 0 in component "Spur Gear (8 teeth)"
sketch "草图2" plane through (0, 0, 0) normal (0, 0, 1) x (1, 0, 0) in component "Spur Gear (8 teeth)"
  spline S0 degree 5 poles (7.3504, -1.5763) (7.3577, -1.5779) (7.3723, -1.5807) (7.3943, -1.5841) (7.4239, -1.5871) (7.4612, -1.5888) (7.4987, -1.5889) (7.5364, -1.588) (7.5741, -1.5866) (7.6119, -1.5849) (7.6498, -1.5827) (7.6877, -1.5801) (7.7257, -1.5767) (7.7638, -1.5726) (7.802, -1.5677) (7.8402, -1.562) (7.8785, -1.5558) (7.9168, -1.549) (7.9551, -1.5418) (7.9935, -1.5341) (8.0319, -1.526) (8.0703, -1.5174) (8.1087, -1.5082) (8.1471, -1.4986) (8.1856, -1.4885) (8.224, -1.4779) (8.2624, -1.4668) (8.3009, -1.4553) (8.3393, -1.4434) (8.3778, -1.4311) (8.4162, -1.4183) (8.4546, -1.4051) (8.4929, -1.3915) (8.5313, -1.3774) (8.5696, -1.363) (8.608, -1.3481) (8.6462, -1.3328) (8.6845, -1.3172) (8.7227, -1.3011) (8.7609, -1.2847) (8.799, -1.2679) (8.8371, -1.2506) (8.8752, -1.2331) (8.9132, -1.2151) (8.9512, -1.1967) (8.9891, -1.178) (9.0269, -1.1589) (9.0647, -1.1395) (9.1025, -1.1197) (9.1401, -1.0995) (9.1778, -1.079) (9.2153, -1.0581) (9.2528, -1.0368) (9.2902, -1.0152) (9.3276, -0.9933) (9.3648, -0.971) (9.402, -0.9484) (9.4392, -0.9254) (9.4762, -0.9021) (9.5132, -0.8784) (9.55, -0.8544) (9.5868, -0.8301) (9.6235, -0.8055) (9.6602, -0.7805) (9.6967, -0.7552) (9.7331, -0.7295) (9.7695, -0.7036) (9.8057, -0.6773) (9.8418, -0.6507) (9.8779, -0.6238) (9.9138, -0.5965) (9.9425, -0.5745) (9.9639, -0.5578) (9.9782, -0.5466) (9.9854, -0.541) knots 0 0 0 0 0 0 0.01428571 0.02857143 0.04285714 0.05714286 0.07142857 0.08571429 0.1 0.11428571 0.12857143 0.14285714 0.15714286 0.17142857 0.18571429 0.2 0.21428571 0.22857143 0.24285714 0.25714286 0.27142857 0.28571429 0.3 0.31428571 0.32857143 0.34285714 0.35714286 0.37142857 0.38571429 0.4 0.41428571 0.42857143 0.44285714 0.45714286 0.47142857 0.48571429 0.5 0.51428571 0.52857143 0.54285714 0.55714286 0.57142857 0.58571429 0.6 0.61428571 0.62857143 0.64285714 0.65714286 0.67142857 0.68571429 0.7 0.71428571 0.72857143 0.74285714 0.75714286 0.77142857 0.78571429 0.8 0.81428571 0.82857143 0.84285714 0.85714286 0.87142857 0.88571429 0.9 0.91428571 0.92857143 0.94285714 0.95714286 0.97142857 0.98571429 1 1 1 1 1 1
  spline S1 degree 5 poles (7.3504, 1.5763) (7.3577, 1.5779) (7.3723, 1.5807) (7.3943, 1.5841) (7.4239, 1.5871) (7.4612, 1.5888) (7.4987, 1.5889) (7.5364, 1.588) (7.5741, 1.5866) (7.6119, 1.5849) (7.6498, 1.5827) (7.6877, 1.5801) (7.7257, 1.5767) (7.7638, 1.5726) (7.802, 1.5677) (7.8402, 1.562) (7.8785, 1.5558) (7.9168, 1.549) (7.9551, 1.5418) (7.9935, 1.5341) (8.0319, 1.526) (8.0703, 1.5174) (8.1087, 1.5082) (8.1471, 1.4986) (8.1856, 1.4885) (8.224, 1.4779) (8.2624, 1.4668) (8.3009, 1.4553) (8.3393, 1.4434) (8.3778, 1.4311) (8.4162, 1.4183) (8.4546, 1.4051) (8.4929, 1.3915) (8.5313, 1.3774) (8.5696, 1.363) (8.608, 1.3481) (8.6462, 1.3328) (8.6845, 1.3172) (8.7227, 1.3011) (8.7609, 1.2847) (8.799, 1.2679) (8.8371, 1.2506) (8.8752, 1.2331) (8.9132, 1.2151) (8.9512, 1.1967) (8.9891, 1.178) (9.0269, 1.1589) (9.0647, 1.1395) (9.1025, 1.1197) (9.1401, 1.0995) (9.1778, 1.079) (9.2153, 1.0581) (9.2528, 1.0368) (9.2902, 1.0152) (9.3276, 0.9933) (9.3648, 0.971) (9.402, 0.9484) (9.4392, 0.9254) (9.4762, 0.9021) (9.5132, 0.8784) (9.55, 0.8544) (9.5868, 0.8301) (9.6235, 0.8055) (9.6602, 0.7805) (9.6967, 0.7552) (9.7331, 0.7295) (9.7695, 0.7036) (9.8057, 0.6773) (9.8418, 0.6507) (9.8779, 0.6238) (9.9138, 0.5965) (9.9425, 0.5745) (9.9639, 0.5578) (9.9782, 0.5466) (9.9854, 0.541) knots 0 0 0 0 0 0 0.01428571 0.02857143 0.04285714 0.05714286 0.07142857 0.08571429 0.1 0.11428571 0.12857143 0.14285714 0.15714286 0.17142857 0.18571429 0.2 0.21428571 0.22857143 0.24285714 0.25714286 0.27142857 0.28571429 0.3 0.31428571 0.32857143 0.34285714 0.35714286 0.37142857 0.38571429 0.4 0.41428571 0.42857143 0.44285714 0.45714286 0.47142857 0.48571429 0.5 0.51428571 0.52857143 0.54285714 0.55714286 0.57142857 0.58571429 0.6 0.61428571 0.62857143 0.64285714 0.65714286 0.67142857 0.68571429 0.7 0.71428571 0.72857143 0.74285714 0.75714286 0.77142857 0.78571429 0.8 0.81428571 0.82857143 0.84285714 0.85714286 0.87142857 0.88571429 0.9 0.91428571 0.92857143 0.94285714 0.95714286 0.97142857 0.98571429 1 1 1 1 1 1
  arc A0 (9.9854, -0.541) -> (9.9854, 0.541) centre (0, 0) ccw
  line L0 (5.4161, -1.1636) -> (7.3504, -1.5763)
  line L1 (5.4161, 1.1636) -> (7.3504, 1.5763)
  line L2 (5.4161, -1.1636) -> (5.4161, 1.1636)
  point P0 (7.5292, -1.5881)
  point P1 (7.7124, -1.5778)
  point P2 (7.8984, -1.5522)
  point P3 (8.0864, -1.5135)
  point P4 (8.2759, -1.4628)
  point P5 (8.4663, -1.4008)
  point P6 (8.6575, -1.3282)
  point P7 (8.8489, -1.2451)
  point P8 (9.0403, -1.152)
  point P9 (9.2313, -1.049)
  point P10 (9.4216, -0.9362)
  point P11 (9.611, -0.8139)
  point P12 (9.799, -0.6821)
  point P13 (7.5292, 1.5881)
  point P14 (7.7124, 1.5778)
  point P15 (7.8984, 1.5522)
  point P16 (8.0864, 1.5135)
  point P17 (8.2759, 1.4628)
  point P18 (8.4663, 1.4008)
  point P19 (8.6575, 1.3282)
  point P20 (8.8489, 1.2451)
  point P21 (9.0403, 1.152)
  point P22 (9.2313, 1.049)
  point P23 (9.4216, 0.9362)
  point P24 (9.611, 0.8139)
  point P25 (9.799, 0.6821)
extrude "拉伸2" add sketch "草图2" along normal blind 5 in component "Spur Gear (8 teeth)"
fillet "圆角1" radius 0.3 2 edges at (5.4254, -1.1656, 2.5) (5.4254, 1.1656, 2.5) in component "Spur Gear (8 teeth)"
pattern_circular "C-阵列1" count 8 over 360 about axis through (0, 0, 0) along (0, 0, 1) of "拉伸2", "圆角1" in component "Spur Gear (8 teeth)"
sketch "草图3" plane through (0, 0, 0) normal (0, 0, 1) x (1, 0, 0) in component "Spur Gear (8 teeth)"
  circle A0 centre (0, 0) radius 8 construction
component "Spur Gear (8 teeth)" placed x (1, 0, 0) y (0, 1, 0) z (0, 0, 1) at (0, 0, 0)

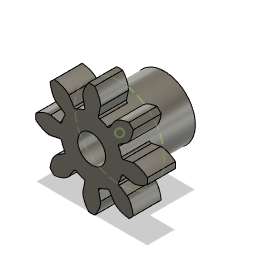
design "gear1245"
description: middle size
description: Spur Gear; Module: 2.0; Num Teeth: 8; Pressure Angle: 20.0; Backlash: 0.00 mm
Autodesk Fusion 360 part; units mm, degrees
sketch "草图1" plane through (0, 0, 0) normal (0, 0, 1) x (1, 0, 0) in component "Spur Gear (8 teeth)"
  circle A0 centre (0, 0) radius 5.5492
  circle A1 centre (0, 0) radius 2.5
extrude "拉伸1" add sketch "草图1" along normal blind 5 and the other way blind 8 in component "Spur Gear (8 teeth)"
sketch "草图2" plane through (0, 0, 0) normal (0, 0, 1) x (1, 0, 0) in component "Spur Gear (8 teeth)"
  spline S0 degree 5 poles (7.3504, -1.5763) (7.3577, -1.5779) (7.3723, -1.5807) (7.3943, -1.5841) (7.4239, -1.5871) (7.4612, -1.5888) (7.4987, -1.5889) (7.5364, -1.588) (7.5741, -1.5866) (7.6119, -1.5849) (7.6498, -1.5827) (7.6877, -1.5801) (7.7257, -1.5767) (7.7638, -1.5726) (7.802, -1.5677) (7.8402, -1.562) (7.8785, -1.5558) (7.9168, -1.549) (7.9551, -1.5418) (7.9935, -1.5341) (8.0319, -1.526) (8.0703, -1.5174) (8.1087, -1.5082) (8.1471, -1.4986) (8.1856, -1.4885) (8.224, -1.4779) (8.2624, -1.4668) (8.3009, -1.4553) (8.3393, -1.4434) (8.3778, -1.4311) (8.4162, -1.4183) (8.4546, -1.4051) (8.4929, -1.3915) (8.5313, -1.3774) (8.5696, -1.363) (8.608, -1.3481) (8.6462, -1.3328) (8.6845, -1.3172) (8.7227, -1.3011) (8.7609, -1.2847) (8.799, -1.2679) (8.8371, -1.2506) (8.8752, -1.2331) (8.9132, -1.2151) (8.9512, -1.1967) (8.9891, -1.178) (9.0269, -1.1589) (9.0647, -1.1395) (9.1025, -1.1197) (9.1401, -1.0995) (9.1778, -1.079) (9.2153, -1.0581) (9.2528, -1.0368) (9.2902, -1.0152) (9.3276, -0.9933) (9.3648, -0.971) (9.402, -0.9484) (9.4392, -0.9254) (9.4762, -0.9021) (9.5132, -0.8784) (9.55, -0.8544) (9.5868, -0.8301) (9.6235, -0.8055) (9.6602, -0.7805) (9.6967, -0.7552) (9.7331, -0.7295) (9.7695, -0.7036) (9.8057, -0.6773) (9.8418, -0.6507) (9.8779, -0.6238) (9.9138, -0.5965) (9.9425, -0.5745) (9.9639, -0.5578) (9.9782, -0.5466) (9.9854, -0.541) knots 0 0 0 0 0 0 0.01428571 0.02857143 0.04285714 0.05714286 0.07142857 0.08571429 0.1 0.11428571 0.12857143 0.14285714 0.15714286 0.17142857 0.18571429 0.2 0.21428571 0.22857143 0.24285714 0.25714286 0.27142857 0.28571429 0.3 0.31428571 0.32857143 0.34285714 0.35714286 0.37142857 0.38571429 0.4 0.41428571 0.42857143 0.44285714 0.45714286 0.47142857 0.48571429 0.5 0.51428571 0.52857143 0.54285714 0.55714286 0.57142857 0.58571429 0.6 0.61428571 0.62857143 0.64285714 0.65714286 0.67142857 0.68571429 0.7 0.71428571 0.72857143 0.74285714 0.75714286 0.77142857 0.78571429 0.8 0.81428571 0.82857143 0.84285714 0.85714286 0.87142857 0.88571429 0.9 0.91428571 0.92857143 0.94285714 0.95714286 0.97142857 0.98571429 1 1 1 1 1 1
  spline S1 degree 5 poles (7.3504, 1.5763) (7.3577, 1.5779) (7.3723, 1.5807) (7.3943, 1.5841) (7.4239, 1.5871) (7.4612, 1.5888) (7.4987, 1.5889) (7.5364, 1.588) (7.5741, 1.5866) (7.6119, 1.5849) (7.6498, 1.5827) (7.6877, 1.5801) (7.7257, 1.5767) (7.7638, 1.5726) (7.802, 1.5677) (7.8402, 1.562) (7.8785, 1.5558) (7.9168, 1.549) (7.9551, 1.5418) (7.9935, 1.5341) (8.0319, 1.526) (8.0703, 1.5174) (8.1087, 1.5082) (8.1471, 1.4986) (8.1856, 1.4885) (8.224, 1.4779) (8.2624, 1.4668) (8.3009, 1.4553) (8.3393, 1.4434) (8.3778, 1.4311) (8.4162, 1.4183) (8.4546, 1.4051) (8.4929, 1.3915) (8.5313, 1.3774) (8.5696, 1.363) (8.608, 1.3481) (8.6462, 1.3328) (8.6845, 1.3172) (8.7227, 1.3011) (8.7609, 1.2847) (8.799, 1.2679) (8.8371, 1.2506) (8.8752, 1.2331) (8.9132, 1.2151) (8.9512, 1.1967) (8.9891, 1.178) (9.0269, 1.1589) (9.0647, 1.1395) (9.1025, 1.1197) (9.1401, 1.0995) (9.1778, 1.079) (9.2153, 1.0581) (9.2528, 1.0368) (9.2902, 1.0152) (9.3276, 0.9933) (9.3648, 0.971) (9.402, 0.9484) (9.4392, 0.9254) (9.4762, 0.9021) (9.5132, 0.8784) (9.55, 0.8544) (9.5868, 0.8301) (9.6235, 0.8055) (9.6602, 0.7805) (9.6967, 0.7552) (9.7331, 0.7295) (9.7695, 0.7036) (9.8057, 0.6773) (9.8418, 0.6507) (9.8779, 0.6238) (9.9138, 0.5965) (9.9425, 0.5745) (9.9639, 0.5578) (9.9782, 0.5466) (9.9854, 0.541) knots 0 0 0 0 0 0 0.01428571 0.02857143 0.04285714 0.05714286 0.07142857 0.08571429 0.1 0.11428571 0.12857143 0.14285714 0.15714286 0.17142857 0.18571429 0.2 0.21428571 0.22857143 0.24285714 0.25714286 0.27142857 0.28571429 0.3 0.31428571 0.32857143 0.34285714 0.35714286 0.37142857 0.38571429 0.4 0.41428571 0.42857143 0.44285714 0.45714286 0.47142857 0.48571429 0.5 0.51428571 0.52857143 0.54285714 0.55714286 0.57142857 0.58571429 0.6 0.61428571 0.62857143 0.64285714 0.65714286 0.67142857 0.68571429 0.7 0.71428571 0.72857143 0.74285714 0.75714286 0.77142857 0.78571429 0.8 0.81428571 0.82857143 0.84285714 0.85714286 0.87142857 0.88571429 0.9 0.91428571 0.92857143 0.94285714 0.95714286 0.97142857 0.98571429 1 1 1 1 1 1
  arc A0 (9.9854, -0.541) -> (9.9854, 0.541) centre (0, 0) ccw
  line L0 (5.4161, -1.1636) -> (7.3504, -1.5763)
  line L1 (5.4161, 1.1636) -> (7.3504, 1.5763)
  line L2 (5.4161, -1.1636) -> (5.4161, 1.1636)
  point P0 (7.5292, -1.5881)
  point P1 (7.7124, -1.5778)
  point P2 (7.8984, -1.5522)
  point P3 (8.0864, -1.5135)
  point P4 (8.2759, -1.4628)
  point P5 (8.4663, -1.4008)
  point P6 (8.6575, -1.3282)
  point P7 (8.8489, -1.2451)
  point P8 (9.0403, -1.152)
  point P9 (9.2313, -1.049)
  point P10 (9.4216, -0.9362)
  point P11 (9.611, -0.8139)
  point P12 (9.799, -0.6821)
  point P13 (7.5292, 1.5881)
  point P14 (7.7124, 1.5778)
  point P15 (7.8984, 1.5522)
  point P16 (8.0864, 1.5135)
  point P17 (8.2759, 1.4628)
  point P18 (8.4663, 1.4008)
  point P19 (8.6575, 1.3282)
  point P20 (8.8489, 1.2451)
  point P21 (9.0403, 1.152)
  point P22 (9.2313, 1.049)
  point P23 (9.4216, 0.9362)
  point P24 (9.611, 0.8139)
  point P25 (9.799, 0.6821)
extrude "拉伸2" add sketch "草图2" along normal blind 5 in component "Spur Gear (8 teeth)"
fillet "圆角1" radius 0.3 2 edges at (5.4254, -1.1656, 2.5) (5.4254, 1.1656, 2.5) in component "Spur Gear (8 teeth)"
pattern_circular "C-阵列1" count 8 over 360 about axis through (0, 0, -8) along (0, 0, 1) of "拉伸2", "圆角1" in component "Spur Gear (8 teeth)"
sketch "草图3" plane through (0, 0, 0) normal (0, 0, 1) x (1, 0, 0) in component "Spur Gear (8 teeth)"
  circle A0 centre (0, 0) radius 8 construction
component "Spur Gear (8 teeth)" placed x (1, 0, 0) y (0, 1, 0) z (0, 0, 1) at (0, 0, 0)

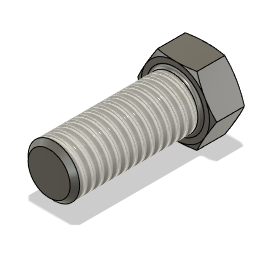
design "bolt"
Autodesk Fusion 360 part; units mm, degrees
sketch "草图1" plane through (0, 0, 0) normal (0, 0, 1) x (1, 0, 0) in component "Component"
  line L0 (1.875, 3.2476) -> (3.75, 0)
  line L1 (-1.875, 3.2476) -> (1.875, 3.2476)
  line L2 (-3.75, 0) -> (-1.875, 3.2476)
  line L3 (-1.875, -3.2476) -> (-3.75, 0)
  line L4 (1.875, -3.2476) -> (-1.875, -3.2476)
  line L5 (3.75, 0) -> (1.875, -3.2476)
extrude "拉伸1" add sketch "草图1" along normal blind 3 in component "Component"
sketch "草图2" plane through (0, 0, 0) normal (0, 0, 1) x (1, 0, 0) in component "Component"
  circle A0 centre (0, 0) radius 2.5
extrude "拉伸2" add sketch "草图2" along normal blind 15 in component "Component"
chamfer "倒角1" distance 0.5 angle 45 1 edges at (-2.3308, -0.904, 15) in component "Component"
fillet "圆角1" radius 0.3 1 edges at (-2.3308, 0.904, 3) in component "Component"
sketch "草图3" plane through (0, 0, 0) normal (0, 1, 0) x (1, 0, 0) in component "Component"
  line L0 (3.2476, 0) -> (3.75, 0)
  line L1 (3.75, 0) -> (3.75, -0.1829)
  line L2 (3.75, -0.1829) -> (3.2476, 0)
  line L3 (3.2476, -3) -> (3.75, -3)
  line L4 (3.75, -3) -> (3.75, -2.8171)
  line L5 (3.75, -2.8171) -> (3.2476, -3)
revolve "旋转1" cut sketch "草图3" angle 360 about axis through (0, 0, 1.75) along (0, 0, 1) contours L3 L4 L5 in component "Component"
revolve "旋转2" cut sketch "草图3" angle 360 about axis through (0, 0, 1.75) along (0, 0, 1) contours L0 L1 L2 in component "Component"
thread "螺纹1" "ISO Metric profile 5.0 M5x0.8 6g" major diameter 4.901 minor diameter 3.9895 pitch 0.8 angle 60 resizes the face on face at (2.4969, -0.1246, 10.7667) in component "Component"
component "Component" placed x (1, 0, 0) y (0, 1, 0) z (0, 0, 1) at (0, 0, 0)
named bodies: "Bolt"

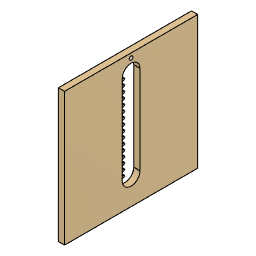
design "extension (up)"
Autodesk Fusion 360 part; units mm, degrees
sketch "Sketch1" plane through (0, 0, 0) normal (0, 1, 0) x (1, 0, 0)
  line L0 (-7, 150) -> (0, 150)
  line L1 (0, 150) -> (0, 0)
  line L2 (0, 0) -> (-7, 0)
  line L3 (-7, 0) -> (-7, 150)
  dimension "d1" = 7
  dimension "d2" = 150
  constraint horizontal L0
  constraint vertical L1
  constraint horizontal L2
  constraint vertical L3
  constraint coincident L1.end L2.start
  measures "d1" distance of L0.start L0.end
  measures "d2" distance of L0.end L1.end
extrude "Extrude1" add sketch "Sketch1" along normal blind 100 and the other way blind 50 makes body 1